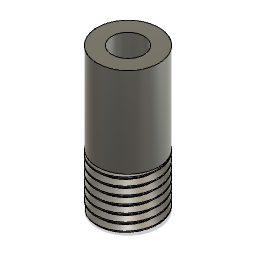
Mic Insert v3 (Autodesk Fusion 360 design; units mm, degrees)
Autodesk Fusion 360 part; units mm, degrees
sketch "Sketch1" plane through (0, 0, 0) normal (0, 0, 1) x (1, 0, 0)
  line L0 (4.14, 0) -> (8, 0)
  line L1 (8, 0) -> (8, 36)
  line L2 (8, 36) -> (4, 36)
  line L3 (4, 36) -> (4, 10.3)
  line L4 (4, 10.3) -> (3.35, 10.3)
  line L5 (3.35, 10.3) -> (4.14, 0)
  line L6 (0, 14.5) -> (0, -2.5)
  dimension "d4" = 10.3
  dimension "d6" = 3.35
  dimension "d7" = 4.14
  dimension "d8" = 4
  dimension "d9" = 36
  dimension "d10" = 8
  constraint horizontal L0
  constraint perpendicular L0 L1
  constraint perpendicular L1 L2
  constraint perpendicular L2 L3
  constraint perpendicular L3 L4
  constraint vertical L6
  measures "d4" distance of L0 L4
  measures "d6" distance of L4.end L6
  measures "d7" distance of L0.start L6
  measures "d8" distance of L3 L6
  measures "d9" distance of L0 L2
  measures "d10" distance of L1 L6
revolve "Revolve1" add sketch "Sketch1" angle 360 about axis through (0, 14.5, 0) along (0, -1, 0)
thread "Thread1" "ISO Metric profile 16.0 M16x2 6g" major diameter 15.822 minor diameter 13.534 pitch 2 angle 60 modelled right hand crest width 0.2847 on face at (7.9602, 24, -0.7965) from (0, 13, 0) to (0, 0, 0) crest through (7.911, 36.5, 0)
move_face "OffsetFaces1" offset -0.1 1 faces at (3.9801, 27.4333, -0.3983)
